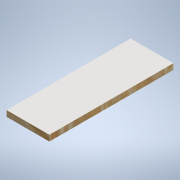
# Autodesk Inventor part: Arm Rest
Saved by Autodesk Inventor 2021.1 (Build 251245000, 245)
## iProperties
Created: 2020-08-02
Part Number: Arm Rest
Material: Wood (Birch)
Document SubType Name: Modeling
Designer: adick
Density: 0.55 g/cm^3
Appearance: Birch - Natural Polished
Author: adick
Autodesk Inventor part; units mm, degrees
ref_plane "YZ Plane" through (0, 0, 0) normal (1, 0, 0) x (0, 1, 0)
ref_plane "XZ Plane" through (0, 0, 0) normal (0, 1, 0) x (-1, 0, 0)
ref_plane "XY Plane" through (0, 0, 0) normal (0, 0, 1) x (1, 0, 0)
sketch "Sketch1" plane through (0, 0, 0) normal (0, 0, 1) x (1, 0, 0)
  line L0 (-135, -7) -> (-35.423, -7) projected
  line L1 (-128.65, -70.65) -> (-128.65, -7) projected
  line L2 (135, -70.65) -> (-135, -70.65) projected
  line L3 (-128.65, -7) -> (-35.423, -7)
  line L4 (-35.423, -7) -> (-35.423, -13.3614)
  line L5 (-35.423, -13.3614) -> (-128.65, -13.3614)
  line L6 (-128.65, -13.3614) -> (-128.65, -7)
  point P0 (0, 0)
  constraints: 8 end point, 2 parallel, 1 horizontal, 1 perpendicular
extrude "Extrusion1" add sketch "Sketch1" along normal blind 270
sketch "Sketch2" plane through (-128.65, -7, 0) normal (0, 1, 0) x (1, 0, 0)
  line L0 (93.227, -270) -> (0, -270) projected
  line L1 (93.227, 0) -> (0, 0) projected
  line L2 (0, -270) -> (93.227, -270)
  line L3 (93.227, -270) -> (93.227, 0)
  line L4 (93.227, 0) -> (0, 0)
  line L5 (0, 0) -> (0, -270)
  point P0 (128.65, 0)
  constraints: 8 end point, 2 parallel, 1 horizontal, 1 perpendicular
extrude "Extrusion2" add sketch "Sketch2" along normal blind 6.35
sketch "Sketch3" plane through (-128.65, -13.3614, 0) normal (-1, 0, 0) x (0, 0, 1)
  line L0 (0, 0) -> (270, 0) projected
  line L1 (0, 0) -> (0, 12.7114) projected
  line L2 (270, 0) -> (0, 0)
  line L3 (0, 0) -> (0, 12.7114)
  line L4 (0, 12.7114) -> (270, 12.7114)
  line L5 (270, 12.7114) -> (270, 0)
  point P0 (0, 13.3614)
  constraints: 8 end point, 2 parallel, 1 horizontal, 1 perpendicular
extrude "Extrusion3" add sketch "Sketch3" along normal blind 12.7
body "Solid1"
